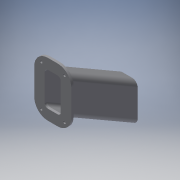
# Autodesk Inventor part: handle
Saved by Autodesk Inventor 2017 (Build 210142000, 142)
## iProperties
Created: 2017-09-05
Part Number: handle
Material: Generic
Document SubType Name: Modeling
Designer: Hp
Density: 1 g/cm^3
Appearance: Default
Author: Hp
Autodesk Inventor part; units mm, degrees
ref_plane "YZ Plane" through (0, 0, 0) normal (1, 0, 0) x (0, 1, 0)
ref_plane "XZ Plane" through (0, 0, 0) normal (0, 1, 0) x (-1, 0, 0)
ref_plane "XY Plane" through (0, 0, 0) normal (0, 0, 1) x (1, 0, 0)
sketch "Sketch1" plane through (0, 0, 0) normal (0, 0, 1) x (1, 0, 0)
  line L0 (7, 0) -> (19, 0)
  line L1 (26, 7) -> (26, 41)
  line L2 (19, 48) -> (7, 48)
  line L3 (0, 41) -> (0, 7)
  arc A0 (7, 48) -> (0, 41) centre (7, 41) ccw
  arc A1 (26, 41) -> (19, 48) centre (19, 41) ccw
  arc A2 (19, 0) -> (26, 7) centre (19, 7) ccw
  arc A3 (0, 7) -> (7, 0) centre (7, 7) ccw
  line L4 (7, 45) -> (19, 45)
  arc A4 (23, 41) -> (19, 45) centre (19, 41) ccw
  line L5 (23, 41) -> (23, 7)
  arc A5 (19, 3) -> (23, 7) centre (19, 7) ccw
  line L6 (19, 3) -> (7, 3)
  arc A6 (3, 7) -> (7, 3) centre (7, 7) ccw
  line L7 (3, 7) -> (3, 41)
  arc A7 (7, 45) -> (3, 41) centre (7, 41) ccw
  point P0 (0, 0)
  point P1 (26, 48)
  point P2 (26, 0)
  point P3 (0, 48)
  dimension "d0" = 26
  dimension "d1" = 48
  dimension "d2" = 7
  dimension "d3" = 3
  constraints: 16 end point, 16 point on circle, 8 centre point, 8 point on line, 8 tangent, 4 parallel, 3 equal radius, 2 perpendicular, 1 horizontal, 7 other
  measures "d0" distance of point (0, 48) point (26, 48)
  measures "d1" distance of point (26, 48) point (26, 0)
  measures "d2" radius of A0
  measures "d3" distance between parallel lines of L7 L3
sketch "Sketch2" plane through (0, 0, 0) normal (1, 0, 0) x (0, 1, 0)
  line L0 (0, 0) -> (0, 90) construction
  line L1 (0, 0) -> (51.9615, 90)
  line L2 (51.9615, 90) -> (0, 90) construction
  dimension "d5" = 90
  dimension "d6" = 30
  constraints: 7 end point, 1 perpendicular, 1 vertical
  measures "d5" distance of L0.start L0.end
  measures "d6" angle of L0 L1
sweep "Sweep1" add profiles "Sketch1" path "Sketch2"
sketch "Sketch4" plane through (7, 99.9615, 90) normal (0, 0, 1) x (1, 0, 0)
  arc A0 (16, -7) -> (12, -3) centre (12, -7) ccw projected
  line L0 (16, -7) -> (16, -41) projected
  arc A1 (12, -45) -> (16, -41) centre (12, -41) ccw projected
  line L1 (12, -45) -> (0, -45) projected
  arc A2 (-4, -41) -> (0, -45) centre (0, -41) ccw projected
  line L2 (-4, -41) -> (-4, -7) projected
  arc A3 (0, -3) -> (-4, -7) centre (0, -7) ccw projected
  line L3 (0, -3) -> (12, -3) projected
  line L4 (12, 0) -> (0, 0) projected
  arc A4 (0, 0) -> (-7, -7) centre (0, -7) ccw projected
  line L5 (-7, -7) -> (-7, -41) projected
  arc A5 (-7, -41) -> (0, -48) centre (0, -41) ccw projected
  line L6 (0, -48) -> (12, -48) projected
  arc A6 (12, -48) -> (19, -41) centre (12, -41) ccw projected
  line L7 (19, -41) -> (19, -7) projected
  arc A7 (19, -7) -> (12, 0) centre (12, -7) ccw projected
  line L8 (-17, -41) -> (-17, -7)
  arc A8 (0, 10) -> (-17, -7) centre (0, -7) ccw
  line L9 (0, 10) -> (12, 10)
  arc A9 (29, -7) -> (12, 10) centre (12, -7) ccw
  line L10 (29, -7) -> (29, -41)
  arc A10 (12, -58) -> (29, -41) centre (12, -41) ccw
  line L11 (12, -58) -> (0, -58)
  arc A11 (-17, -41) -> (0, -58) centre (0, -41) ccw
  line L12 (-8.4853, -49.4853) -> (-12.0208, -53.0208) construction
  line L13 (-8.4853, -49.4853) -> (-4.9497, -45.9497) construction
  arc A12 (-7, -41) -> (0, -48) centre (0, -41) ccw construction
  line L14 (-4.9497, -45.9497) -> (0, -41) construction
  line L15 (0, -7) -> (-4.9497, -2.0503) construction
  line L16 (-8.4853, 1.4853) -> (-12.0208, 5.0208) construction
  line L17 (-8.4853, 1.4853) -> (-4.9497, -2.0503) construction
  line L18 (12, -7) -> (16.9497, -2.0503) construction
  line L19 (16.9497, -2.0503) -> (20.4853, 1.4853) construction
  line L20 (20.4853, 1.4853) -> (24.0208, 5.0208) construction
  line L21 (12, -41) -> (16.9497, -45.9497) construction
  arc A13 (12, -48) -> (19, -41) centre (12, -41) ccw construction
  line L22 (16.9497, -45.9497) -> (20.4853, -49.4853) construction
  line L23 (20.4853, -49.4853) -> (24.0208, -53.0208) construction
  line L24 (0, -54.9615) -> (0, -3) construction
  line L25 (12, -54.9615) -> (12, -3) construction
  circle A14 centre (20.4853, 1.4853) radius 3
  circle A15 centre (-8.4853, 1.4853) radius 3
  circle A16 centre (-8.4853, -49.4853) radius 3
  circle A17 centre (20.4853, -49.4853) radius 3
  point P0 (-7, -99.9615)
  dimension "d12" = 10
  dimension "d51" = 45
  dimension "d53" = 45
  dimension "d54" = 45
  dimension "d55" = 45
  dimension "d66" = 6
  dimension "d67" = 6
  dimension "d68" = 6
  dimension "d69" = 6
  constraints: 32 end point, 18 point on circle, 10 collinear, 8 centre point, 4 coincident, 4 line through centre, 7 other
  measures "d12" distance between parallel lines of L5 L8
  measures "d51" angle of L2 L14
  measures "d53" angle of L24 L15
  measures "d54" angle of L25 L18
  measures "d55" angle of L25 L21
  measures "d66" diameter of A14
  measures "d67" diameter of A15
  measures "d68" diameter of A16
  measures "d69" diameter of A17
extrude "Extrusion1" add sketch "Sketch4" along normal blind 3 contours A7 L7 A6 L6 A5 L5 A4 L4 | L8 A8 L9 A9 L10 A10 L11 A11 | A14 | A15 | A16 | A17
fillet "Fillet1" radius 8 8 edges at (0, 75.9615, 90) (2.0503, 54.0118, 90) (13, 51.9615, 90) (23.9497, 54.0118, 90) (26, 75.9615, 90) (23.9497, 97.9113, 90) (13, 99.9615, 90) (2.0503, 97.9113, 90)
hole "Hole1" at (-1.4853, 50.4762, 90) at (-1.4853, 101.4468, 90) at (27.4853, 101.4468, 90) at (27.4853, 50.4762, 90) direction (0, 0, 1) diameter 3.25 end through all countersink diameter 6 countersink angle 90
extrude "Extrusion2" cut sketch "Sketch4" against normal blind 6 contours A14 | A15 | A16 | A17
equation "\"d53\" = d51"
equation "\"d54\" = d51"
equation "\"d55\" = d51"
body "Solid1"
